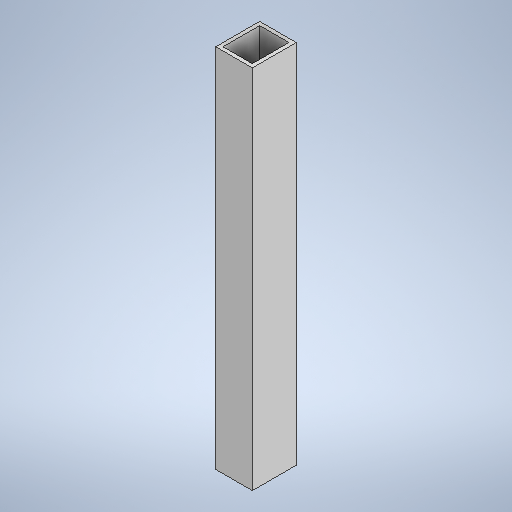
# Autodesk Inventor part: 25 cm trunk
Saved by Autodesk Inventor 2025 (Build 290162000, 162)
## iProperties
Created: 2024-07-29
Part Number: 25 cm trunk
Material: Generic
Document SubType Name: Modeling
Designer: Isaac
Density: 1 g/cm^3
Appearance: Default
Author: Isaac
Autodesk Inventor part; units mm, degrees
ref_plane "YZ Plane" through (0, 0, 0) normal (1, 0, 0) x (0, 1, 0)
ref_plane "XZ Plane" through (0, 0, 0) normal (0, 1, 0) x (-1, 0, 0)
ref_plane "XY Plane" through (0, 0, 0) normal (0, 0, 1) x (1, 0, 0)
sketch "Sketch1" plane through (0, 0, 0) normal (0, 1, 0) x (-1, 0, 0)
  line L0 (-12.5, 15) -> (12.5, 15)
  line L1 (12.5, 15) -> (12.5, -15)
  line L2 (12.5, -15) -> (-12.5, -15)
  line L3 (-12.5, -15) -> (-12.5, 15)
  line L4 (-12.5, 15) -> (12.5, -15) construction
  line L5 (12.5, 15) -> (-12.5, -15) construction
  point P0 (0, 0)
  dimension "d0" = 30
  dimension "d1" = 25
  constraints: 12 end point, 2 midpoint, 2 parallel, 1 horizontal, 1 perpendicular
  measures "d0" distance of L0.end L1.end
  measures "d1" distance of L1.end L2.end
extrude "Extrusion1" add sketch "Sketch1" along normal blind 250
sketch "Sketch2" plane through (0, 250, 0) normal (0, 1, 0) x (1, 0, 0)
  line L0 (-10, -12.5) -> (10, -12.5)
  line L1 (10, -12.5) -> (10, 12.5)
  line L2 (10, 12.5) -> (-10, 12.5)
  line L3 (-10, 12.5) -> (-10, -12.5)
  line L4 (-10, -12.5) -> (10, 12.5) construction
  line L5 (10, -12.5) -> (-10, 12.5) construction
  point P0 (0, 0)
  dimension "d4" = 25
  dimension "d5" = 20
  constraints: 12 end point, 2 midpoint, 2 parallel, 1 horizontal, 1 perpendicular
  measures "d4" distance of L0.end L1.end
  measures "d5" distance of L1.end L2.end
extrude "Extrusion2" cut sketch "Sketch2" against normal blind 600
body "Solid1"
